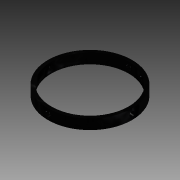
# Autodesk Inventor part: Ball Ring
Saved by Autodesk Inventor 2013 (Build 170138000, 138)
## iProperties
Created: 2012-09-25
Part Number: Ball Ring
Material: Generic
Document SubType Name: Modeling
Designer: uqgtayle
Density: 1 g/cm^3
Author: uqgtayle
Autodesk Inventor part; units mm, degrees
ref_plane "YZ Plane" through (0, 0, 0) normal (1, 0, 0) x (0, 1, 0)
sketch "Sketch1" plane through (0, 0, 0) normal (0, 0, 1) x (1, 0, 0)
  circle A0 centre (0, 0) radius 23
  circle A1 centre (0, 0) radius 25
  dimension "d0" = 50
  dimension "d2" = 46
  constraints: 2 centre point, 2 coincident
  measures "d0" diameter of A1
  measures "d2" diameter of A0
extrude "Extrusion1" add sketch "Sketch1" against normal blind 6
sketch "Sketch2" plane through (0, 0, 0) normal (0, 1, 0) x (-1, 0, 0)
  line L0 (-25, -6) -> (25, -6) projected
  circle A0 centre (0, -3) radius 1.5
  point P0 (0, 0)
  dimension "d5" = 3
  dimension "d6" = 3
  constraints: 1 centre point, 1 coincident
  measures "d5" distance from line of L0 point (0, -3)
  measures "d6" diameter of A0
extrude "Extrusion2" cut sketch "Sketch2" along normal through all both and the other way through all
sketch "Sketch3" plane through (0, 0, 0) normal (1, 0, 0) x (0, 1, 0)
  circle A0 centre (0, -3) radius 1.5
  line L0 (-25, 0) -> (25, 0) projected
  point P0 (0, 0)
  dimension "d9" = 3
  dimension "d10" = 3
  constraints: 1 centre point
  measures "d9" distance from line of L0 A0.centre
  measures "d10" diameter of A0
extrude "Extrusion3" cut sketch "Sketch3" along normal through all both and the other way through all
ref_plane "Work Plane1" through (0, 0, 0) normal (0.4226, 0.9063, 0) x (0, 0, -1)
ref_plane "Work Plane2" through (10.5655, 22.6577, 0) normal (0.4226, 0.9063, 0) x (0, 0, -1)
sketch "Sketch5" plane through (10.5655, 22.6577, 0) normal (0.4226, 0.9063, 0) x (0, 0, -1)
  circle A0 centre (3, 0) radius 1.5
  line L0 (0, 25) -> (6, 25) projected
  point P0 (0, 0)
  point P1 (3, 25)
  dimension "d17" = 3
  constraints: 1 centre point, 1 midpoint, 1 vertical alignment
  measures "d17" diameter of A0
extrude "Extrusion4" cut sketch "Sketch5" against normal blind 10
body "Solid1"
